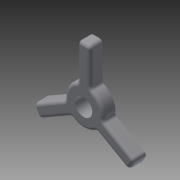
# Autodesk Inventor part: ALLIGNER
Saved by Autodesk Inventor 2013 (Build 170138000, 138)
## iProperties
Created: 2013-12-04
Part Number: ALLIGNER
Material: Generic
Document SubType Name: Modeling
Designer: employee
Density: 1 g/cm^3
Author: employee
Autodesk Inventor part; units mm, degrees
ref_plane "YZ Plane" through (0, 0, 0) normal (1, 0, 0) x (0, 1, 0)
ref_plane "XZ Plane" through (0, 0, 0) normal (0, 1, 0) x (-1, 0, 0)
ref_plane "XY Plane" through (0, 0, 0) normal (0, 0, 1) x (1, 0, 0)
sketch "Sketch1" plane through (0, 0, 0) normal (0, 0, 1) x (1, 0, 0)
  circle A0 centre (0, 0) radius 4.0687
  arc A1 (-3, 8.5582) -> (3, 8.5582) centre (0, 0) ccw
  arc A2 (3, 26.0022) -> (-3, 26.0022) centre (0, 0) ccw
  line L0 (-3, 8.5582) -> (-3, 26.0022)
  line L1 (3, 8.5582) -> (3, 26.0022)
  dimension "d0" = 26.1747
  dimension "d2" = 6
  dimension "d3" = 5
  dimension "d4" = 8.1375
  constraints: 4 end point, 4 point on circle, 3 centre point, 3 coincident, 2 parallel, 1 vertical
  measures "d0" radius of A2
  measures "d2" distance between parallel lines of L1 L0
  measures "d3" radial gap between concentric circles of A1 A0
  measures "d4" diameter of A0
extrude "Extrusion1" add sketch "Sketch1" along normal blind 6
pattern_circular "Circular Pattern1" count 3 over 360 about axis through (0, 0, 0) along (0, 0, 1) of "Extrusion1"
fillet "Fillet1" radius 1.5875 24 edges at (-5.9116, -6.8772, 3) (5.9116, -6.8772, 3) (8.9116, -1.681, 3) (3, 8.5582, 3) (-3, 8.5582, 3) (-8.9116, -1.681, 3) (-21.0186, -15.5992, 3) (-24.0186, -10.403, 3) (-3, 26.0022, 3) (3, 26.0022, 3) (21.0186, -15.5992, 3) (24.0186, -10.403, 3) (-22.668, -13.0874, 6) (0, 26.1747, 6) (22.668, -13.0874, 6) (-13.4651, -11.2382, 6) (0, -9.0687, 6) (13.4651, -11.2382, 6) (16.4651, -6.042, 6) (7.8538, 4.5344, 6) (3, 17.2802, 6) (-3, 17.2802, 6) (-7.8538, 4.5344, 6) (-16.4651, -6.042, 6)
body "Solid1"
